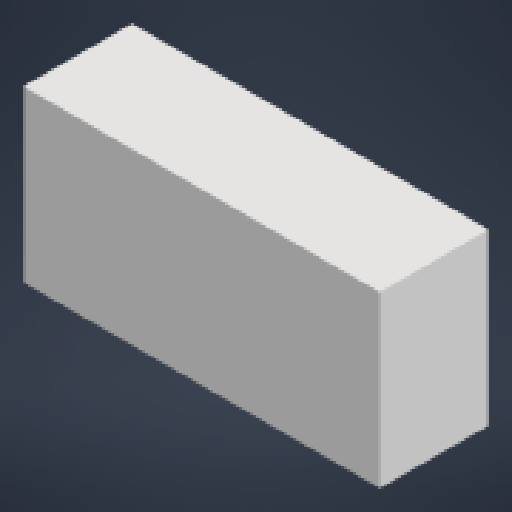
# Autodesk Inventor part: PJ-242
Saved by Autodesk Inventor 2023 (Build 270158000, 158)
## iProperties
Created: 2022-10-25
Part Number: PJ-242
Material: Generic
Document SubType Name: Modeling
Designer: jevan
Density: 1 g/cm^3
Appearance: Default
Author: jevan
Autodesk Inventor part; units mm, degrees
ref_plane "YZ Plane" through (0, 0, 0) normal (1, 0, 0) x (0, 1, 0)
ref_plane "XZ Plane" through (0, 0, 0) normal (0, 1, 0) x (-1, 0, 0)
ref_plane "XY Plane" through (0, 0, 0) normal (0, 0, 1) x (1, 0, 0)
sketch "Sketch1" plane through (0, 0, 0) normal (0, 0, 1) x (1, 0, 0)
  line L0 (0, 0) -> (10.5, 0)
  line L1 (10.5, 0) -> (10.5, -5)
  line L2 (10.5, -5) -> (0, -5)
  line L3 (0, -5) -> (0, 0)
  dimension "d0" = 10.5
  dimension "d1" = 5
  constraints: 8 end point, 2 parallel, 1 horizontal, 1 perpendicular
  measures "d0" distance of L1.end L2.end
  measures "d1" distance of L0.end L1.end
extrude "Extrusion1" add sketch "Sketch1" along normal blind 3.2
sketch "Sketch2" plane through (0, -5, 0) normal (-1, 0, 0) x (0, 0, 1)
  line L0 (0, 0) -> (0, 5) projected
  line L1 (0, 2.5) -> (1.6, 2.5)
  circle A0 centre (1.6, 2.5) radius 1.3
  circle A1 centre (1.6, 2.5) radius 2
  point P0 (0, 1.3)
  point P1 (0, 3.7)
  dimension "d4" = 1.6
  dimension "d5" = 2.6
  dimension "d6" = 4
  constraints: 2 centre point, 2 coincident, 2 end point, 1 horizontal, 1 midpoint
  measures "d4" distance of L1.start L1.end
  measures "d5" diameter of A0
  measures "d6" diameter of A1
extrude "Extrusion2" add sketch "Sketch2" along normal blind 1.5
extrude "Extrusion3" cut sketch "Sketch2" against normal through all contours A0
move faces "Move1" translate (-0.7, 0, 0) faces at (0, -2.7773, 3.2729)
sketch "Sketch3" plane through (0, 0, 0) normal (0, 0, -1) x (-1, 0, 0)
  line L0 (0, 0) -> (0, -5) projected
  line L1 (0, -5) -> (0, 0)
  line L2 (0, -2.5) -> (-9.1, -2.5)
  line L3 (-9.1, -2.5) -> (-9.1, -5.6)
  line L4 (-9.1, -5.6) -> (-8.6, -5.6)
  line L5 (-9.1, -5.6) -> (-9.6, -5.6)
  line L6 (-9.6, -5.6) -> (-9.6, -5)
  line L7 (0, -5) -> (-10.5, -5) projected
  line L8 (-8.6, -5.6) -> (-8.6, -5)
  line L9 (-9.6, -5) -> (-8.6, -5)
  line L10 (-9.1, -5) -> (-5.4, -5)
  line L11 (-5.4, -5) -> (-4.9, -5)
  line L12 (-4.9, -5) -> (-4.9, -5.6)
  line L13 (-4.9, -5.6) -> (-5.9, -5.6)
  line L14 (-5.9, -5.6) -> (-5.9, -5)
  line L15 (-5.4, -5) -> (-1.7, -5)
  line L16 (-1.7, -5) -> (-1.2, -5)
  line L17 (-1.2, -5) -> (-1.2, -5.6)
  line L18 (-1.2, -5.6) -> (-2.2, -5.6)
  line L19 (-2.2, -5.6) -> (-2.2, -5)
  line L20 (-9.1, 0.6) -> (-8.6, 0.6)
  line L21 (-9.1, 0.6) -> (-9.6, 0.6)
  line L22 (-9.6, 0.6) -> (-9.6, 0)
  line L23 (-8.6, 0.6) -> (-8.6, 0)
  line L24 (-9.6, 0) -> (-8.6, 0)
  line L25 (-9.1, 0) -> (-5.4, 0)
  line L26 (-5.4, 0) -> (-4.9, 0)
  line L27 (-4.9, 0) -> (-4.9, 0.6)
  line L28 (-4.9, 0.6) -> (-5.9, 0.6)
  line L29 (-5.9, 0.6) -> (-5.9, 0)
  line L30 (-5.4, 0) -> (-1.7, 0)
  line L31 (-1.7, 0) -> (-1.2, 0)
  line L32 (-1.2, 0) -> (-1.2, 0.6)
  line L33 (-1.2, 0.6) -> (-2.2, 0.6)
  line L34 (-2.2, 0.6) -> (-2.2, 0)
  point P0 (0, -3.7)
  dimension "d14" = 9.1
  dimension "d15" = 3.1
  dimension "d16" = 0.5
  dimension "d17" = 0.5
  dimension "d18" = 3.7
  dimension "d19" = 0.5
  dimension "d20" = 1
  dimension "d21" = 3.7
  dimension "d22" = 0.5
  dimension "d23" = 1
  constraints: 66 end point, 16 point on line, 16 symmetric about line, 6 perpendicular, 3 horizontal, 2 midpoint, 2 vertical, 1 collinear, 1 parallel
  measures "d14" distance of L2.start L2.end
  measures "d15" distance of L2.end L3.end
  measures "d16" distance of L3.end L4.end
  measures "d17" distance of L3.end L5.end
  measures "d18" distance of L10.start L10.end
  measures "d19" distance of L10.end L11.end
  measures "d20" distance of L12.end L13.end
  measures "d21" distance of L10.end L15.end
  measures "d22" distance of L15.end L16.end
  measures "d23" distance of L17.end L18.end
extrude "Extrusion4" add sketch "Sketch3" against normal blind 0.1 contours L17 L18 L19 L7 | L7 L8 L4 L3 | L3 L5 L6 L7 | L7 L12 L13 L14 | L20 L23 L24 L22 L21 | L29 L28 L27 L26 L25 | L34 L33 L32 L31 L30
body "Solid1"
